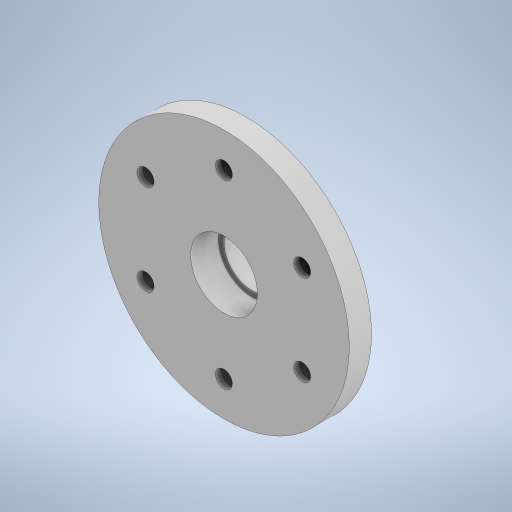
# Autodesk Inventor part: Input pin holder
Saved by Autodesk Inventor 2023 (Build 270158000, 158)
## iProperties
Created: 2023-01-17
Part Number: Input pin holder
Material: Generic
Document SubType Name: Modeling
Designer: caden
Density: 1 g/cm^3
Appearance: Default
Mass: 54.0244 g
Surface Area: 184.78 cm^2
Volume: 54.0244 cm^3
Author: caden
Autodesk Inventor part; units mm, degrees
ref_plane "YZ Plane" through (0, 0, 0) normal (1, 0, 0) x (0, 1, 0)
ref_plane "XZ Plane" through (0, 0, 0) normal (0, 1, 0) x (-1, 0, 0)
ref_plane "XY Plane" through (0, 0, 0) normal (0, 0, 1) x (1, 0, 0)
ref_plane "Work Plane1" through (0, 0, 2.9972) normal (0, 0, 1) x (1, 0, 0)
sketch "Sketch1" plane through (0, 0, 2.9972) normal (0, 0, 1) x (1, 0, 0)
  circle A0 centre (0, 0) radius 17.4625
  circle A1 centre (0, 0) radius 32.5 construction
  circle A2 centre (0, 0) radius 45
  circle A3 centre (0, -32.5) radius 4.5
  circle A4 centre (28.1458, -16.25) radius 4.5
  circle A5 centre (28.1458, 16.25) radius 4.5
  circle A6 centre (0, 32.5) radius 4.5
  circle A7 centre (-28.1458, 16.25) radius 4.5
  circle A8 centre (-28.1458, -16.25) radius 4.5
  point P0 (0, 0)
  dimension "d1" = 65
  dimension "d0" = 34.925
  dimension "d2" = 90
  dimension "d3" = 9
  dimension "d6" = 360
  constraints: 8 centre point, 3 coincident, 1 vertical alignment, 15 other
  measures "d0" diameter of A0
  measures "d2" diameter of A2
  measures "d3" diameter of A3
extrude "Extrusion1" add sketch "Sketch1" along normal blind 8 contours A0 | A2
ref_plane "Work Plane2" through (-75, -75, -12) normal (0, 0, -1) x (0, 1, 0)
extrude "Extrusion2" add sketch "Sketch1" against normal up to surface (14.9972 mm away) contours A0
sketch "Sketch3" plane through (0, 0, 10.9972) normal (0, 0, 1) x (1, 0, 0)
  circle A0 centre (-28.1458, -16.25) radius 4.5 projected
  circle A1 centre (-28.1458, -16.25) radius 3
  circle A2 centre (0, 32.5) radius 4.5 projected
  circle A3 centre (0, 32.5) radius 3
  circle A4 centre (-28.1458, 16.25) radius 4.5 projected
  circle A5 centre (-28.1458, 16.25) radius 3
  circle A6 centre (28.1458, 16.25) radius 4.5 projected
  circle A7 centre (28.1458, 16.25) radius 3
  circle A8 centre (28.1458, -16.25) radius 4.5 projected
  circle A9 centre (28.1458, -16.25) radius 3
  circle A10 centre (0, -32.5) radius 4.5 projected
  circle A11 centre (0, -32.5) radius 3
  point P0 (0, 0)
  dimension "d12" = 6
  dimension "d13" = 6
  dimension "d14" = 6
  dimension "d15" = 6
  dimension "d16" = 6
  dimension "d17" = 6
  constraints: 6 centre point, 6 coincident
  measures "d12" diameter of A1
  measures "d13" diameter of A3
  measures "d14" diameter of A5
  measures "d15" diameter of A7
  measures "d16" diameter of A9
  measures "d17" diameter of A11
extrude "Extrusion3" add sketch "Sketch3" against normal blind 2
sketch "Sketch4" plane through (0, 0, 10.9972) normal (0, 0, 1) x (1, 0, 0)
  point P0 (0, 0)
  point P1 (0, 0)
  constraints: 1 coincident
hole "Hole1" at (0, 0, 10.9972) direction (0, 0, -1) diameter 20 end through all counterbore diameter 24 counterbore depth 10
sketch "Sketch5" plane through (0, 0, 2.9972) normal (0, 0, -1) x (-1, 0, 0)
  circle A0 centre (0, 0) radius 15.7248
  circle A1 centre (0, 0) radius 18.2248
  circle A2 centre (0, 0) radius 17.4625 projected
  point P0 (0, 0)
  dimension "d27" = 2.5
  constraints: 2 centre point, 2 coincident
  measures "d27" radial gap between concentric circles of A1 A0
extrude "Extrusion4" add sketch "Sketch5" along normal blind 1 contours A1
body "Solid1"
